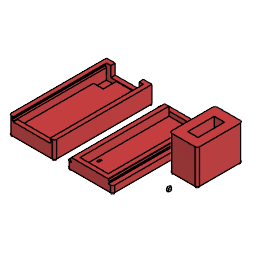
red_ducky-case (Autodesk Fusion 360 design; units mm, degrees)
part number: 2025-12-17-15-00-24-933
part number: 2025-12-19-11-25-16-273
Autodesk Fusion 360 part; units mm, degrees
note: some values were not read from the file. Chosen so that the rebuilt part matches the saved one: which face or edge a step refers to; which pieces of a blend or face edit are solid. Set by a fixed rule: which sketch regions a step uses.
sketch "Sketch1" plane through (0, 0, 0) normal (1, 0, 0) x (0, 1, 0)
  line L0 (-7.5042, 20.5557) -> (9.4958, 20.5557)
  line L1 (9.4958, 20.5557) -> (9.4958, -20.4443)
  line L2 (9.4958, -20.4443) -> (-7.5042, -20.4443)
  line L3 (-7.5042, -20.4443) -> (-7.5042, 20.5557)
  line L4 (-9.5042, 22.5557) -> (11.4958, 22.5557)
  line L5 (11.4958, 22.5557) -> (11.4958, -22.4443)
  line L6 (11.4958, -22.4443) -> (-9.5042, -22.4443)
  line L7 (-9.5042, -22.4443) -> (-9.5042, 22.5557)
  line L8 (-7.5042, 20.5557) -> (-3.0042, 20.5557)
  line L9 (-3.0042, 20.5557) -> (-3.0042, 14.5557)
  line L10 (-3.0042, 14.5557) -> (-7.5042, 14.5557)
  line L11 (-7.5042, 14.5557) -> (-7.5042, 20.5557)
  line L12 (9.4958, 20.5557) -> (4.9958, 20.5557)
  line L13 (4.9958, 20.5557) -> (4.9958, 14.5557)
  line L14 (4.9958, 14.5557) -> (9.4958, 14.5557)
  line L15 (9.4958, 14.5557) -> (9.4958, 20.5557)
  dimension "d1" = 17
  dimension "d2" = 41
  dimension "d3" = 45
  dimension "d4" = 21
  dimension "d5" = 2
  dimension "d6" = 2
  dimension "d8" = 6
  dimension "d9" = 4.5
  dimension "d10" = 6
  dimension "d11" = 4.5
  constraint horizontal L0
  constraint vertical L1
  constraint horizontal L2
  constraint vertical L3
  constraint horizontal L4
  constraint vertical L5
  constraint horizontal L6
  constraint vertical L7
  constraint horizontal L8
  constraint vertical L9
  constraint horizontal L10
  constraint vertical L11
  constraint horizontal L12
  constraint vertical L13
  constraint horizontal L14
  constraint vertical L15
  measures "d1" distance of L1 L3
  measures "d2" distance of L0 L2
  measures "d3" distance of L4.start L6.end
  measures "d4" distance of L4.start L4.end
  measures "d5" distance of L3 L7
  measures "d6" distance of L0 L4
  measures "d8" distance of L0.start L10.end
  measures "d9" distance of L9 L11
  measures "d10" distance of L0.end L14.end
  measures "d11" distance of L13 L15
extrude "Extrude1" add sketch "Sketch1" along normal blind 2 contours L0 L3 L8 L9 L10 L11 | L0 L1 L12 L13 L14 L15 makes body 1 at (0, -6.0042, 16.5557) makes body 2 at (0, 7.9958, 16.5557)
extrude "Extrude2" add sketch "Sketch1" along normal blind 4 contours L0 L1 L2 L3 L9 L10 L13 L14 bodies 1 2
extrude "Extrude3" add sketch "Sketch1" along normal blind 10.8 bodies 1
sketch "Sketch2" plane through (10.8, 0, 0) normal (1, 0, 0) x (0, 1, 0)
  line L0 (9.4958, 20.5557) -> (9.4958, -20.4443)
  line L1 (9.4958, -20.4443) -> (-7.5042, -20.4443)
  line L2 (-7.5042, -20.4443) -> (-7.5042, 20.5557)
  line L3 (-7.5042, 20.5557) -> (9.4958, 20.5557)
  line L4 (-9.5042, -22.4443) -> (11.4958, -22.4443)
  line L5 (11.4958, -22.4443) -> (11.4958, 22.5557)
  line L6 (11.4958, 22.5557) -> (-9.5042, 22.5557)
  line L7 (-9.5042, 22.5557) -> (-9.5042, -22.4443)
  line L8 (-6.5042, 22.5557) -> (8.4958, 22.5557)
  line L9 (8.4958, 22.5557) -> (8.4958, 20.5557)
  line L10 (8.4958, 20.5557) -> (-6.5042, 20.5557)
  line L11 (-6.5042, 20.5557) -> (-6.5042, 22.5557)
  line L12 (11.4958, 22.5557) -> (11.4958, -22.4443)
  dimension "d18" = 15
  dimension "d19" = 3
  constraint horizontal L8
  constraint vertical L9
  constraint horizontal L10
  constraint vertical L11
  constraint coincident L3 L9.end
  constraint coincident L6 L8.start
  measures "d18" distance of L9 L11
  measures "d19" distance of L9 L12
extrude "Extrude4" cut sketch "Sketch2" against normal blind 2 contours L0 L1 L2 L3 L4 L5 L6 L7 L9 L11 L12 | L3 L6 L8 L9 L10 L11 bodies 1
extrude "Extrude5" cut sketch "Sketch2" against normal blind 5 contours L3 L6 L8 L9 L10 L11 bodies 1
extrude "Extrude6" cut 1 faces at (5.8, 3.4958, 21.2224) along direction (-1, 0, 0) blind 2 on bodies 1 bodies 1
extrude "Extrude7" add 1 faces at (5.4667, -6.5042, 21.8891) along direction (0, 1, 0) blind 1 on bodies 1 bodies 1
extrude "Extrude8" add 1 faces at (7.1333, 8.4958, 21.8891) along direction (0, -1, 0) blind 1 on bodies 1 bodies 1
sketch "Sketch3" plane through (0, 0, -22.4443) normal (0, 0, -1) x (1, 0, 0)
  line L0 (8.8, -11.4958) -> (8.8, 9.5042)
  line L1 (8.8, 9.5042) -> (0, 9.5042)
  line L2 (0, 9.5042) -> (0, -11.4958)
  line L3 (0, -11.4958) -> (8.8, -11.4958)
  line L4 (8.8, 9.5042) -> (0, 9.5042)
  line L5 (0, 9.5042) -> (0, 7.5042)
  line L6 (0, 7.5042) -> (8.8, 7.5042)
  line L7 (8.8, 7.5042) -> (8.8, 9.5042)
  line L8 (8.8, -11.4958) -> (0, -11.4958)
  line L9 (0, -11.4958) -> (0, -9.4958)
  line L10 (0, -9.4958) -> (8.8, -9.4958)
  line L11 (8.8, -9.4958) -> (8.8, -11.4958)
  line L12 (8.8, 7.5042) -> (6.8, 7.5042)
  line L13 (6.8, 7.5042) -> (6.8, -9.4958)
  line L14 (6.8, -9.4958) -> (8.8, -9.4958)
  line L15 (8.8, -9.4958) -> (8.8, 7.5042)
  line L16 (8.05, 7.5042) -> (7.55, 7.5042)
  line L17 (7.5494, 8.0042) -> (8.05, 8.0042)
  line L18 (8.05, 8.0042) -> (8.55, 7.5042)
  line L19 (7.5494, 8.0042) -> (7.0494, 7.5042)
  line L20 (8.05, -9.4958) -> (7.55, -9.4958)
  line L21 (7.55, -9.9958) -> (8.05, -9.9958)
  line L22 (8.05, -9.9958) -> (8.5529, -9.4929)
  line L23 (7.55, -9.9958) -> (7.05, -9.4958)
  dimension "d30" = 2
  dimension "d31" = 2
  dimension "d32" = 2
  dimension "d33" = 0.5
  dimension "d36" = 0.5
  dimension "d39" = 45
  dimension "d40" = 45
  dimension "d41" = 45
  dimension "d42" = 45
  constraint horizontal L4
  constraint vertical L5
  constraint horizontal L6
  constraint vertical L7
  constraint coincident L2 L5.end
  constraint coincident L0.end L1.start
  constraint horizontal L8
  constraint vertical L9
  constraint horizontal L10
  constraint vertical L11
  constraint coincident L2 L9.end
  constraint coincident L0.start L3.end
  constraint horizontal L12
  constraint vertical L13
  constraint horizontal L14
  constraint vertical L15
  constraint coincident L10 L13.end
  constraint horizontal L16
  constraint horizontal L17
  constraint coincident L6 L16.start
  constraint coincident L6 L18.end
  constraint coincident L6 L19.end
  constraint horizontal L20
  constraint horizontal L21
  constraint coincident L14 L20.start
  constraint coincident L14 L23.end
  measures "d30" distance of L0.end L6.end
  measures "d31" distance of L0.start L10.end
  measures "d32" distance of L13 L15
  measures "d33" distance of L16.start L17.end
  measures "d36" distance of L20.start L21.end
  measures "d39" angle of L10 L22
  measures "d40" angle of L12 L18
  measures "d41" angle of L12 L19
  measures "d42" angle of L14 L23
extrude "Extrude9" cut sketch "Sketch3" against normal blind 2 contours L0 L6 L10 L12 L13 L14 L15 L16 L20 bodies 1
extrude "Extrude10" cut sketch "Sketch3" against normal blind 43 contours L10 L14 L20 L21 L22 L23 | L6 L12 L16 L17 L18 L19 bodies 1
extrude "Extrude11" add 1 faces at (3.8, -0.3375, 21.8891) along direction (1, 0, 0) blind 0.2 on bodies 1 bodies 1
sketch "Sketch4" plane through (0, 9.9958, 0) normal (0, -1, 0) x (1, 0, 0)
  line L0 (7.55, -22.4443) -> (8.05, -22.4443)
  line L1 (8.05, -22.4443) -> (8.05, 20.5557)
  line L2 (8.05, 20.5557) -> (7.55, 20.5557)
  line L3 (7.55, 20.5557) -> (7.55, -22.4443)
  line L4 (7.55, 20.5557) -> (8.05, 20.5557)
  line L5 (8.05, 20.5557) -> (8.05, 20.0557)
  line L6 (8.05, 20.0557) -> (7.55, 20.0557)
  line L7 (8.05, 20.0557) -> (8.05, 18.5557)
  line L8 (8.05, 18.5557) -> (7.55, 18.5557)
  line L9 (7.55, 18.5557) -> (7.55, 20.0557)
  dimension "d49" = 0.5
  dimension "d50" = 1.5
  constraint horizontal L4
  constraint vertical L5
  constraint horizontal L6
  constraint coincident L2.end L3.start
  constraint vertical L7
  constraint horizontal L8
  constraint vertical L9
  measures "d49" distance of L2.end L6.end
  measures "d50" distance of L6.end L8.end
extrude "Extrude12" cut sketch "Sketch4" against normal blind 1 contours L1 L2 L3 L4 L5 L6 bodies 1
chamfer "Chamfer1" distance 1.5 distance2 1 1 edges at (7.8, 9.9958, 20.0557) measured on face at (7.7167, 9.9958, -8.2776) on bodies 1
sketch "Sketch5" plane through (0, -8.0042, 0) normal (0, 1, 0) x (-1, 0, 0)
  line L0 (-8.05, -22.4443) -> (-7.5494, -22.4443)
  line L1 (-7.5494, -22.4443) -> (-7.5494, 20.5557)
  line L2 (-7.5494, 20.5557) -> (-8.05, 20.5557)
  line L3 (-8.05, 20.5557) -> (-8.05, -22.4443)
  line L4 (-8.05, 20.5557) -> (-7.5494, 20.5557)
  line L5 (-7.5494, 20.5557) -> (-7.5494, 20.0557)
  line L6 (-7.5494, 20.0557) -> (-8.05, 20.0557)
  line L7 (-8.05, 20.0557) -> (-8.05, 20.5557)
  line L8 (-8.05, 20.0557) -> (-7.5, 20.0557)
  line L9 (-7.5, 20.0557) -> (-7.5, 18.5557)
  line L10 (-7.5, 18.5557) -> (-8.05, 18.5557)
  line L11 (-8.05, 18.5557) -> (-8.05, 20.0557)
  dimension "d55" = 0.5
  dimension "d56" = 1.5
  constraint horizontal L4
  constraint vertical L5
  constraint horizontal L6
  constraint vertical L7
  constraint coincident L2.end L3.start
  constraint horizontal L8
  constraint vertical L9
  constraint horizontal L10
  constraint vertical L11
  measures "d55" distance of L2.end L6.end
  measures "d56" distance of L6.end L10.end
extrude "Extrude13" cut sketch "Sketch5" against normal blind 1 contours L1 L2 L3 L4 L5 L6 L7 L8 bodies 1
chamfer "Chamfer2" distance 1.5 distance2 1 1 edges at (7.7997, -8.0042, 20.0557) measured on face at (7.8831, -8.0042, -8.2776) on bodies 1
sketch "Sketch6" plane through (0, 0, 0) normal (1, 0, 0) x (0, 1, 0)
  line L0 (24.8147, 22.7428) -> (45.8147, 22.7428)
  line L1 (45.8147, 22.7428) -> (45.8147, -22.2572)
  line L2 (45.8147, -22.2572) -> (24.8147, -22.2572)
  line L3 (24.8147, -22.2572) -> (24.8147, 22.7428)
  dimension "d65" = 45
  dimension "d73" = 21
  constraint horizontal L0
  constraint vertical L1
  constraint horizontal L2
  constraint vertical L3
  measures "d65" distance of L0.start L2.end
  measures "d73" distance of L1 L3
extrude "Extrude16" add sketch "Sketch6" along normal blind 2 separate body makes body 3
sketch "Sketch7" plane through (2, 0, 0) normal (1, 0, 0) x (0, 1, 0)
  line L0 (24.8147, -22.2572) -> (45.8147, -22.2572)
  line L1 (45.8147, -22.2572) -> (45.8147, 22.7428)
  line L2 (45.8147, 22.7428) -> (24.8147, 22.7428)
  line L3 (24.8147, 22.7428) -> (24.8147, -22.2572)
  line L4 (24.8147, 22.7428) -> (45.8147, 22.7428)
  line L5 (45.8147, 22.7428) -> (45.8147, 20.7428)
  line L6 (45.8147, 20.7428) -> (24.8147, 20.7428)
  line L7 (24.8147, 20.7428) -> (24.8147, 22.7428)
  line L8 (45.8147, 22.7428) -> (43.8147, 22.7428)
  line L9 (43.8147, 22.7428) -> (43.8147, -22.2572)
  line L10 (43.8147, -22.2572) -> (45.8147, -22.2572)
  line L11 (45.8147, -22.2572) -> (45.8147, 22.7428)
  line L12 (24.8147, -22.2572) -> (45.8147, -22.2572)
  line L13 (45.8147, -22.2572) -> (45.8147, -20.2572)
  line L14 (45.8147, -20.2572) -> (24.8147, -20.2572)
  line L15 (24.8147, -20.2572) -> (24.8147, -22.2572)
  line L16 (24.8147, -22.2572) -> (26.8147, -22.2572)
  line L17 (26.8147, -22.2572) -> (26.8147, 23)
  line L18 (26.8147, 23) -> (24.8147, 23)
  line L19 (24.8147, 23) -> (24.8147, -22.2572)
  line L20 (26.8147, 20.7428) -> (28.8147, 20.7428)
  line L21 (28.8147, 20.7428) -> (28.8147, -22.2572)
  line L22 (28.8147, -22.2572) -> (26.8147, -22.2572)
  line L23 (26.8147, -22.2572) -> (26.8147, 20.7428)
  line L24 (43.8147, 20.7428) -> (41.8147, 20.7428)
  line L25 (41.8147, 20.7428) -> (41.8147, -22.2572)
  line L26 (41.8147, -22.2572) -> (43.8147, -22.2572)
  line L27 (43.8147, -22.2572) -> (43.8147, 20.7428)
  dimension "d76" = 2
  dimension "d77" = 2
  dimension "d78" = 2
  dimension "d79" = 2
  dimension "d80" = 2
  dimension "d81" = 2
  constraint horizontal L4
  constraint vertical L5
  constraint horizontal L6
  constraint vertical L7
  constraint coincident L2.end L3.start
  constraint horizontal L8
  constraint vertical L9
  constraint horizontal L10
  constraint vertical L11
  constraint coincident L0 L9.end
  constraint coincident L1.end L2.start
  constraint horizontal L12
  constraint vertical L13
  constraint horizontal L14
  constraint vertical L15
  constraint coincident L0.start L3.end
  constraint horizontal L16
  constraint vertical L17
  constraint horizontal L18
  constraint vertical L19
  constraint horizontal L20
  constraint vertical L21
  constraint horizontal L22
  constraint vertical L23
  constraint coincident L12 L21.end
  constraint coincident L17 L20.start
  constraint coincident L6 L20.start
  constraint horizontal L24
  constraint vertical L25
  constraint horizontal L26
  constraint vertical L27
  constraint coincident L0 L25.end
  constraint coincident L9 L24.start
  constraint coincident L6 L24.start
  measures "d76" distance of L2.end L6.end
  measures "d77" distance of L9 L11
  measures "d78" distance of L0.start L14.end
  measures "d79" distance of L17 L19
  measures "d80" distance of L17 L21
  measures "d81" distance of L9 L25
extrude "Extrude17" add sketch "Sketch7" along normal blind 2 contours L0 L3 L12 L14 L15 L16 L17 L19 L23 | L3 L6 L14 L17 L19 L23 | L2 L3 L4 L6 L7 L17 L19 | L2 L4 L6 L9 L17 L20 L24 | L0 L1 L9 L10 L11 L12 L13 L14 L27 | L1 L6 L9 L11 L14 L27 | L1 L2 L4 L5 L6 L8 L9 L11 bodies 3
extrude "Extrude18" add sketch "Sketch7" along normal blind 4 contours L0 L12 L14 L17 L21 L22 L23 | L0 L12 L14 L21 L25 | L6 L14 L17 L20 L21 L23 | L0 L9 L12 L14 L25 L26 L27 | L6 L9 L14 L24 L25 L27 bodies 3
sketch "Sketch8" plane through (0, 26.8147, 0) normal (0, -1, 0) x (1, 0, 0)
  line L0 (4, 20.7428) -> (4, -22.2572)
  line L1 (4, -22.2572) -> (6, -22.2572)
  line L2 (6, -22.2572) -> (6, 20.7428)
  line L3 (6, 20.7428) -> (4, 20.7428)
  line L4 (6, 20.7428) -> (5.75, 20.7428)
  line L5 (5.75, 20.7428) -> (5.75, -22.2572)
  line L6 (5.75, -22.2572) -> (6, -22.2572)
  line L7 (6, -22.2572) -> (6, 20.7428)
  line L8 (5.75, 20.7428) -> (5.25, 20.7428)
  line L9 (5.25, 20.7428) -> (5.25, -22.2572)
  line L10 (5.25, -22.2572) -> (5.75, -22.2572)
  line L11 (5.75, -22.2572) -> (5.75, 20.7428)
  line L12 (5.25, 20.7428) -> (4.75, 20.7428)
  line L13 (4.75, 20.7428) -> (4.75, -22.2572)
  line L14 (4.75, -22.2572) -> (5.25, -22.2572)
  line L15 (5.25, -22.2572) -> (5.25, 20.7428)
  line L16 (4, 20.7428) -> (4.25, 20.7428)
  line L17 (4.25, 20.7428) -> (4.25, -22.2572)
  line L18 (4.25, -22.2572) -> (4, -22.2572)
  line L19 (4, -22.2572) -> (4, 20.7428)
  dimension "d86" = 0.25
  dimension "d87" = 0.5
  dimension "d88" = 0.5
  dimension "d89" = 0.25
  constraint horizontal L4
  constraint vertical L5
  constraint horizontal L6
  constraint vertical L7
  constraint coincident L1 L5.end
  constraint coincident L2.end L3.start
  constraint horizontal L8
  constraint vertical L9
  constraint horizontal L10
  constraint vertical L11
  constraint coincident L1 L9.end
  constraint horizontal L12
  constraint vertical L13
  constraint horizontal L14
  constraint vertical L15
  constraint coincident L1 L13.end
  constraint horizontal L16
  constraint vertical L17
  constraint horizontal L18
  constraint vertical L19
  constraint coincident L1 L17.end
  constraint coincident L0.start L3.end
  measures "d86" distance of L5 L7
  measures "d87" distance of L5 L9
  measures "d88" distance of L9 L13
  measures "d89" distance of L17 L19
extrude "Extrude19" add sketch "Sketch8" along normal blind 0.5 contours L1 L3 L9 L12 L13 L14 L15 bodies 3
extrude "Extrude20" add sketch "Sketch8" along normal blind 0.5 contours L1 L3 L13 L17 | L1 L3 L5 L8 L9 L10 L11 L15 bodies 3
chamfer "Chamfer3" distance 0.5 angle 45 2 edges at (5.75, 26.3147, -0.7572) (4.25, 26.3147, -0.7572) on bodies 3
extrude "Extrude21" add 1 faces at (7.7167, 10.9958, 20.3891) along direction (0, -1, 0) blind 0.5 on bodies 1 bodies 1
delete_face "DeleteFace1" 5 faces at (7.8833, 10.829, 20.0557) (7.8833, 10.6623, 19.5558) (7.55, 10.1625, 19.7225) (7.7167, 10.4958, 20.3891) (8.05, 10.1625, 19.7225) on bodies 1
extrude "Extrude22" cut sketch "Sketch4" against normal blind 0.5 contours L1 L2 L3 L4 L5 L6 bodies 1
chamfer "Chamfer4" distance 1.5 distance2 0.5 1 edges at (7.8, 9.9958, 20.0557) measured on face at (7.7167, 9.9958, -8.2776) on bodies 1
delete_face "DeleteFace2" 5 faces at (8.05, -8.3375, 19.7225) (7.8831, -8.3375, 19.0559) (7.5494, -8.3375, 19.7225) (7.8831, -9.0042, 20.3891) (7.7163, -9.0041, 20.0557) on bodies 1
extrude "Extrude23" cut sketch "Sketch5" against normal blind 0.5 contours L1 L2 L3 L4 L5 L6 L7 L8 bodies 1
chamfer "Chamfer5" distance 1.5 distance2 0.5 1 edges at (7.7997, -8.0042, 20.0557) measured on face at (7.8831, -8.0042, -8.2776) on bodies 1
sketch "Sketch9" plane through (0, 26.3147, 0) normal (0, -1, 0) x (1, 0, 0)
  line L0 (4.75, 20.7428) -> (4.75, -22.2572)
  line L1 (4.75, -22.2572) -> (5.25, -22.2572)
  line L2 (5.25, -22.2572) -> (5.25, 20.7428)
  line L3 (5.25, 20.7428) -> (4.75, 20.7428)
  line L4 (4.75, 20.7428) -> (5.25, 20.7428)
  line L5 (5.25, 20.7428) -> (5.25, 19.2428)
  line L6 (5.25, 19.2428) -> (4.75, 19.2428)
  line L7 (4.75, 19.2428) -> (4.75, 20.7428)
  line L8 (4.75, 19.2428) -> (5.25, 19.2428)
  line L9 (5.25, 19.2428) -> (5.25, 18.7428)
  line L10 (5.25, 18.7428) -> (4.75, 18.7428)
  line L11 (4.75, 18.7428) -> (4.75, 19.2428)
  line L12 (4.75, 18.7428) -> (5.25, 18.7428)
  line L13 (5.25, 18.7428) -> (5.25, 17.2428)
  line L14 (5.25, 17.2428) -> (4.75, 17.2428)
  line L15 (4.75, 17.2428) -> (4.75, 18.7428)
  dimension "d105" = 1.5
  dimension "d106" = 0.5
  dimension "d107" = 1.5
  constraint horizontal L4
  constraint vertical L5
  constraint horizontal L6
  constraint vertical L7
  constraint coincident L0.start L3.end
  constraint horizontal L8
  constraint vertical L9
  constraint horizontal L10
  constraint vertical L11
  constraint horizontal L12
  constraint vertical L13
  constraint horizontal L14
  constraint vertical L15
  measures "d105" distance of L0.start L6.end
  measures "d106" distance of L6.end L10.end
  measures "d107" distance of L10.end L14.end
extrude "Extrude24" add sketch "Sketch9" along normal blind 0.5 contours L0 L2 L6 L8 L9 L10 L11 L12 bodies 3
chamfer "Chamfer6" distance 1.5 distance2 0.5 1 edges at (5, 26.3147, 18.7428) measured on face at (5.0833, 26.3147, -8.5905) on bodies 3
chamfer "Chamfer7" distance 1.5 distance2 0.5 1 edges at (5, 26.3147, 19.2428) measured on face at (5.0833, 26.3147, -9.0904) on bodies 3
sketch "Sketch10" plane through (0, 43.8147, 0) normal (0, 1, 0) x (-1, 0, 0)
  line L0 (-4, -22.2572) -> (-4, 20.7428)
  line L1 (-4, 20.7428) -> (-6, 20.7428)
  line L2 (-6, 20.7428) -> (-6, -22.2572)
  line L3 (-6, -22.2572) -> (-4, -22.2572)
  line L4 (-6, 20.7428) -> (-5.75, 20.7428)
  line L5 (-5.75, 20.7428) -> (-5.75, -22.2572)
  line L6 (-5.75, -22.2572) -> (-6, -22.2572)
  line L7 (-6, -22.2572) -> (-6, 20.7428)
  line L8 (-4, -22.2572) -> (-4.25, -22.2572)
  line L9 (-4.25, -22.2572) -> (-4.25, 20.7428)
  line L10 (-4.25, 20.7428) -> (-4, 20.7428)
  line L11 (-4, 20.7428) -> (-4, -22.2572)
  line L12 (-5.75, -22.2572) -> (-5.25, -22.2572)
  line L13 (-5.25, -22.2572) -> (-5.25, 20.7428)
  line L14 (-5.25, 20.7428) -> (-5.75, 20.7428)
  line L15 (-5.75, 20.7428) -> (-5.75, -22.2572)
  line L16 (-5.25, -22.2572) -> (-4.75, -22.2572)
  line L17 (-4.75, -22.2572) -> (-4.75, 20.7428)
  line L18 (-4.75, 20.7428) -> (-5.25, 20.7428)
  line L19 (-5.25, 20.7428) -> (-5.25, -22.2572)
  dimension "d114" = 0.25
  dimension "d115" = 0.25
  dimension "d116" = 0.5
  dimension "d117" = 0.5
  constraint horizontal L4
  constraint vertical L5
  constraint horizontal L6
  constraint vertical L7
  constraint coincident L3 L5.end
  constraint coincident L1.end L2.start
  constraint horizontal L8
  constraint vertical L9
  constraint horizontal L10
  constraint vertical L11
  constraint coincident L1 L9.end
  constraint coincident L0.start L3.end
  constraint horizontal L12
  constraint vertical L13
  constraint horizontal L14
  constraint vertical L15
  constraint coincident L1 L13.end
  constraint horizontal L16
  constraint vertical L17
  constraint horizontal L18
  constraint vertical L19
  constraint coincident L1 L17.end
  measures "d114" distance of L5 L7
  measures "d115" distance of L9 L11
  measures "d116" distance of L5 L13
  measures "d117" distance of L17 L19
extrude "Extrude25" add sketch "Sketch10" along normal blind 0.5 contours L1 L3 L9 L17 | L1 L3 L13 L16 L17 L18 L19 | L1 L3 L5 L12 L13 L14 L15 L19 bodies 3
chamfer "Chamfer8" distance 0.5 distance2 0.5 1 edges at (5.75, 44.3147, -0.7572) measured on face at (4.75, 44.3147, -7.9238) on bodies 3
chamfer "Chamfer9" distance 0.5 distance2 0.5 1 edges at (4.25, 44.3147, -0.7572) measured on face at (4.9167, 44.3147, -7.9238) on bodies 3
sketch "Sketch11" plane through (0, 44.3147, 0) normal (0, 1, 0) x (-1, 0, 0)
  line L0 (-4.75, -22.2572) -> (-4.75, 20.7428)
  line L1 (-4.75, 20.7428) -> (-5.25, 20.7428)
  line L2 (-5.25, 20.7428) -> (-5.25, -22.2572)
  line L3 (-5.25, -22.2572) -> (-4.75, -22.2572)
  line L4 (-5.25, 20.7428) -> (-4.75, 20.7428)
  line L5 (-4.75, 20.7428) -> (-4.75, 19.2428)
  line L6 (-4.75, 19.2428) -> (-5.25, 19.2428)
  line L7 (-5.25, 19.2428) -> (-5.25, 20.7428)
  line L8 (-5.25, 19.2428) -> (-4.75, 19.2428)
  line L9 (-4.75, 19.2428) -> (-4.75, 18.7428)
  line L10 (-4.75, 18.7428) -> (-5.25, 18.7428)
  line L11 (-5.25, 18.7428) -> (-5.25, 19.2428)
  line L12 (-5.25, 18.7428) -> (-4.75, 18.7428)
  line L13 (-4.75, 18.7428) -> (-4.75, 17.2428)
  line L14 (-4.75, 17.2428) -> (-5.25, 17.2428)
  line L15 (-5.25, 17.2428) -> (-5.25, 18.7428)
  dimension "d124" = 1.5
  dimension "d125" = 0.5
  dimension "d126" = 1.5
  constraint horizontal L4
  constraint vertical L5
  constraint horizontal L6
  constraint vertical L7
  constraint coincident L1.end L2.start
  constraint horizontal L8
  constraint vertical L9
  constraint horizontal L10
  constraint vertical L11
  constraint horizontal L12
  constraint vertical L13
  constraint horizontal L14
  constraint vertical L15
  measures "d124" distance of L1.end L6.end
  measures "d125" distance of L6.end L10.end
  measures "d126" distance of L10.end L14.end
extrude "Extrude26" add sketch "Sketch11" along normal blind 0.5 contours L0 L2 L10 L12 L13 L14 L15 | L0 L2 L6 L8 L9 L10 L11 L12 | L0 L1 L2 L4 L5 L6 L7 L8 bodies 3
chamfer "Chamfer10" distance 1.5 distance2 0.5 2 edges at (5, 44.8147, 17.2428) (5, 44.8147, 20.7428) measured on face at (5.0833, 44.8147, 18.4095) measured on face at (5.0833, 44.8147, 18.4095) on bodies 3
delete_face "DeleteFace3" 5 faces at (7.55, 10.1624, 19.7225) (7.7167, 10.1624, 19.0559) (8.05, 10.1624, 19.7225) (7.7167, 10.4958, 20.3891) (7.8833, 10.4957, 20.0557) on bodies 1
sketch "Sketch12" plane through (0, 9.9958, 0) normal (0, -1, 0) x (1, 0, 0)
  line L0 (7.55, 20.5557) -> (7.55, -22.4443)
  line L1 (7.55, -22.4443) -> (8.05, -22.4443)
  line L2 (8.05, -22.4443) -> (8.05, 20.5557)
  line L3 (8.05, 20.5557) -> (7.55, 20.5557)
  line L4 (7.55, 20.5557) -> (8.05, 20.5557)
  line L5 (8.05, 20.5557) -> (8.05, 19.0557)
  line L6 (8.05, 19.0557) -> (7.55, 19.0557)
  line L7 (7.55, 19.0557) -> (7.55, 20.5557)
  line L8 (7.55, 19.0557) -> (8.05, 19.0557)
  line L9 (8.05, 19.0557) -> (8.05, 18.4557)
  line L10 (8.05, 18.4557) -> (7.55, 18.4557)
  line L11 (7.55, 18.4557) -> (7.55, 19.0557)
  line L12 (7.55, 18.4557) -> (8.05, 18.4557)
  line L13 (8.05, 18.4557) -> (8.05, 16.9557)
  line L14 (8.05, 16.9557) -> (7.55, 16.9557)
  line L15 (7.55, 16.9557) -> (7.55, 18.4557)
  dimension "d131" = 1.5
  dimension "d132" = 0.6
  dimension "d133" = 1.5
  constraint horizontal L4
  constraint vertical L5
  constraint horizontal L6
  constraint vertical L7
  constraint coincident L2 L5.end
  constraint coincident L0.start L3.end
  constraint horizontal L8
  constraint vertical L9
  constraint horizontal L10
  constraint vertical L11
  constraint horizontal L12
  constraint vertical L13
  constraint horizontal L14
  constraint vertical L15
  measures "d131" distance of L0.start L6.end
  measures "d132" distance of L6.end L10.end
  measures "d133" distance of L10.end L14.end
extrude "Extrude27" cut sketch "Sketch12" against normal blind 0.5 contours L0 L2 L6 L8 L9 L10 L11 L12 bodies 1
chamfer "Chamfer11" distance 1.5 distance2 0.5 2 edges at (7.8, 9.9958, 18.4557) (7.8, 9.9958, 19.0557) measured on face at (7.7167, 9.9958, -8.8109) measured on face at (7.8833, 9.9958, 20.0557) on bodies 1
delete_face "DeleteFace4" 5 faces at (8.05, -8.1708, 19.7225) (7.8831, -8.1708, 19.0559) (7.5494, -8.1708, 19.7225) (7.8831, -8.5042, 20.3891) (7.7163, -8.5041, 20.0557) on bodies 1
sketch "Sketch13" plane through (0, -8.0042, 0) normal (0, 1, 0) x (-1, 0, 0)
  line L0 (-8.05, 20.5557) -> (-8.05, -22.4443)
  line L1 (-8.05, -22.4443) -> (-7.5494, -22.4443)
  line L2 (-7.5494, -22.4443) -> (-7.5494, 20.5557)
  line L3 (-7.5494, 20.5557) -> (-8.05, 20.5557)
  line L4 (-8.05, 20.5557) -> (-7.5494, 20.5557)
  line L5 (-7.5494, 20.5557) -> (-7.5494, 19.0557)
  line L6 (-7.5494, 19.0557) -> (-8.05, 19.0557)
  line L7 (-8.05, 19.0557) -> (-8.05, 20.5557)
  line L8 (-8.05, 19.0557) -> (-7.5494, 19.0557)
  line L9 (-7.5494, 19.0557) -> (-7.5494, 18.4557)
  line L10 (-7.5494, 18.4557) -> (-8.05, 18.4557)
  line L11 (-8.05, 18.4557) -> (-8.05, 19.0557)
  line L12 (-8.05, 18.4557) -> (-7.5494, 18.4557)
  line L13 (-7.5494, 18.4557) -> (-7.5494, 16.9557)
  line L14 (-7.5494, 16.9557) -> (-8.05, 16.9557)
  line L15 (-8.05, 16.9557) -> (-8.05, 18.4557)
  dimension "d138" = 1.5
  dimension "d139" = 0.6
  dimension "d140" = 1.5
  constraint horizontal L4
  constraint vertical L5
  constraint horizontal L6
  constraint vertical L7
  constraint coincident L0.start L3.end
  constraint horizontal L8
  constraint vertical L9
  constraint horizontal L10
  constraint vertical L11
  constraint horizontal L12
  constraint vertical L13
  constraint horizontal L14
  constraint vertical L15
  measures "d138" distance of L0.start L6.end
  measures "d139" distance of L6.end L10.end
  measures "d140" distance of L10.end L14.end
extrude "Extrude28" cut sketch "Sketch13" against normal blind 0.5 contours L0 L2 L6 L8 L9 L10 L11 L12 bodies 1
chamfer "Chamfer12" distance 1.5 distance2 0.5 2 edges at (7.7997, -8.0042, 19.0557) (7.7997, -8.0042, 18.4557) measured on face at (7.8831, -8.0042, 20.0557) measured on face at (7.7163, -8.0042, -8.8109) on bodies 1
fillet "Fillet1" radius 1 1 edges at (0, 11.4958, 0.0557) on bodies 1
fillet "Fillet2" radius 1 1 edges at (0, -9.5042, 0.0557) on bodies 1
fillet "Fillet3" radius 1 5 edges at (4.9, 11.4958, -22.4443) (0.2929, 11.2029, -22.4443) (0, 0.9958, -22.4443) (0.2929, -9.2113, -22.4443) (4.9, -9.5042, -22.4443) on bodies 1
fillet "Fillet4" radius 1 1 edges at (2, 24.8147, -22.2572) on bodies 3
fillet "Fillet5" radius 1 3 edges at (0, 35.8147, -22.2572) (0, 25.1076, -21.9643) (0, 24.8147, 0.7428) on bodies 3
fillet "Fillet6" radius 1 3 edges at (0, 45.8147, 0.7428) (0.2929, 45.8147, -21.9643) (2.5, 45.8147, -22.2572) on bodies 3
move_body "Move1" bodies 3 to x (-1, 0, 0) y (0, -1, 0) z (0, 0, 1) at (12.8, 36.3294, 0)
move_body "Move2" bodies 3 to x (1, 0, 0) y (0, 1, 0) z (0, 0, 1) at (0, 0, -0.2)
move_body "Move3" bodies 3 to x (1, 0, 0) y (0, 1, 0) z (0, 0, 1) at (0, 0, 0.023)
move_body "Move4" bodies 3 to x (1, 0, 0) y (0, 1, 0) z (0, 0, 1) at (0, -0.019, 0)
move_body "Move5" bodies 3 to x (1, 0, 0) y (0, 1, 0) z (0, 0, 1) at (0, 0, -0.01)
sketch "Sketch14" plane through (4, 0, 0) normal (1, 0, 0) x (0, 1, 0)
  line L0 (-3.0042, 20.5557) -> (-3.0042, 14.5557)
  line L1 (-3.0042, 14.5557) -> (-7.5042, 14.5557)
  line L2 (-7.5042, 14.5557) -> (-7.5042, -20.4443)
  line L3 (-7.5042, -20.4443) -> (9.4958, -20.4443)
  line L4 (9.4958, -20.4443) -> (9.4958, 14.5557)
  line L5 (9.4958, 14.5557) -> (4.9958, 14.5557)
  line L6 (4.9958, 14.5557) -> (4.9958, 20.5557)
  line L7 (4.9958, 20.5557) -> (7.4958, 20.5557)
  line L8 (7.4958, 20.5557) -> (7.4958, 22.5557)
  line L9 (7.4958, 22.5557) -> (-5.5042, 22.5557)
  line L10 (-5.5042, 22.5557) -> (-5.5042, 20.5557)
  line L11 (-5.5042, 20.5557) -> (-3.0042, 20.5557)
  line L12 (7.4958, 20.5557) -> (-5.5042, 20.5557)
  line L13 (-5.5042, 20.5557) -> (-5.5042, 22.5557)
  line L14 (-5.5042, 22.5557) -> (7.4958, 22.5557)
  line L15 (7.4958, 22.5557) -> (7.4958, 20.5557)
  constraint horizontal L12
  constraint vertical L13
  constraint horizontal L14
  constraint vertical L15
  constraint coincident L9.end L10.start
  constraint coincident L7.end L8.start
extrude "Extrude29" cut sketch "Sketch14" against normal blind 0.2 contours L0 L1 L2 L3 L4 L5 L6 L12 bodies 1
extrude "Extrude30" cut 1 faces at (3.8, 2.3291, -8.7776) along direction (-1, 0, 0) blind 0.5 on bodies 1 bodies 1
extrude "Extrude31" add 1 faces at (3.3, 2.3291, -8.7776) along direction (1, 0, 0) blind 0.4 on bodies 1 bodies 1
sketch "Sketch15" plane through (12.8, 0, 0) normal (1, 0, 0) x (0, 1, 0)
  line L0 (-8.5043, 22.5558) -> (-8.5043, -21.4442)
  line L1 (-8.5043, -21.4442) -> (10.4957, -21.4442)
  line L2 (10.4957, -21.4442) -> (10.4957, 22.5558)
  line L3 (10.4957, 22.5558) -> (-8.5043, 22.5558)
  line L4 (-8.5043, -21.4442) -> (10.4957, -21.4442)
  line L5 (10.4957, -21.4442) -> (10.4957, -20.4442)
  line L6 (10.4957, -20.4442) -> (-8.5043, -20.4442)
  line L7 (-8.5043, -20.4442) -> (-8.5043, -21.4442)
  line L8 (-8.5043, 22.5558) -> (10.4957, 22.5558)
  line L9 (10.4957, 22.5558) -> (10.4957, 20.5558)
  line L10 (10.4957, 20.5558) -> (-8.5043, 20.5558)
  line L11 (-8.5043, 20.5558) -> (-8.5043, 22.5558)
  line L12 (-8.5043, 22.5558) -> (-7.5043, 22.5558)
  line L13 (-7.5043, 22.5558) -> (-7.5043, -21.4442)
  line L14 (-7.5043, -21.4442) -> (-8.5043, -21.4442)
  line L15 (-8.5043, -21.4442) -> (-8.5043, 22.5558)
  line L16 (10.4957, 22.5558) -> (9.4957, 22.5558)
  line L17 (9.4957, 22.5558) -> (9.4957, -21.4442)
  line L18 (9.4957, -21.4442) -> (10.4957, -21.4442)
  line L19 (10.4957, -21.4442) -> (10.4957, 22.5558)
  line L20 (5.3957, -12.4442) -> (6.1957, -12.4442)
  line L21 (6.1957, -12.4442) -> (6.1957, -14.0442)
  line L22 (6.1957, -14.0442) -> (5.3957, -14.0442)
  line L23 (5.3957, -14.0442) -> (5.3957, -12.4442)
  dimension "d163" = 1
  dimension "d164" = 2
  dimension "d165" = 1
  dimension "d166" = 1
  dimension "d167" = 17
  dimension "d168" = 6.4
  dimension "d169" = 3.3
  dimension "d170" = 0.8
  dimension "d171" = 1.6
  constraint horizontal L4
  constraint vertical L5
  constraint horizontal L6
  constraint vertical L7
  constraint coincident L0.end L1.start
  constraint horizontal L8
  constraint vertical L9
  constraint horizontal L10
  constraint vertical L11
  constraint coincident L0.start L3.end
  constraint horizontal L12
  constraint vertical L13
  constraint horizontal L14
  constraint vertical L15
  constraint coincident L4 L13.end
  constraint horizontal L16
  constraint vertical L17
  constraint horizontal L18
  constraint vertical L19
  constraint coincident L4 L17.end
  constraint horizontal L20
  constraint vertical L21
  constraint horizontal L22
  constraint vertical L23
  measures "d163" distance of L0.end L6.end
  measures "d164" distance of L0.start L10.end
  measures "d165" distance of L13 L15
  measures "d166" distance of L17 L19
  measures "d167" distance of L13 L17
  measures "d168" distance of L6 L22
  measures "d169" distance of L17 L21
  measures "d170" distance of L21 L23
  measures "d171" distance of L20 L22
extrude "Extrude32" cut sketch "Sketch15" against normal blind 2 contours L20 L21 L22 L23 bodies 3
extrude "Extrude1'" add 1 faces at (12.1333, 6.1957, -12.9775) along direction (0, -1, 0) blind 0.8 separate body on bodies 3 makes body 4 in component "LED_hole"
extrude "Extrude2'" cut 1 faces at (10.8, 5.929, -12.9775) along direction (1, 0, 0) blind 0.5 on bodies 4 bodies 4 in component "LED_hole"
sketch "Sketch16" plane through (0, 0, 0) normal (0, 0, 1) x (1, 0, 0)
  line L0 (0.1176, 41.5067) -> (12.9176, 41.5067)
  line L1 (12.9176, 41.5067) -> (12.9176, 20.5067)
  line L2 (12.9176, 20.5067) -> (0.1176, 20.5067)
  line L3 (0.1176, 20.5067) -> (0.1176, 41.5067)
  dimension "d178" = 12.8
  dimension "d179" = 21
  constraint horizontal L0
  constraint vertical L1
  constraint horizontal L2
  constraint vertical L3
  measures "d178" distance of L1 L3
  measures "d179" distance of L0 L2
extrude "Extrude33" add sketch "Sketch16" along normal blind 2 separate body makes body 5
sketch "Sketch17" plane through (0, 0, 2) normal (0, 0, 1) x (-1, 0, 0)
  line L0 (-0.1176, -20.5067) -> (-12.9176, -20.5067)
  line L1 (-12.9176, -20.5067) -> (-12.9176, -41.5067)
  line L2 (-12.9176, -41.5067) -> (-0.1176, -41.5067)
  line L3 (-0.1176, -41.5067) -> (-0.1176, -20.5067)
  line L4 (-4.1676, -37.1067) -> (-8.8676, -37.1067)
  line L5 (-8.8676, -37.1067) -> (-8.8676, -24.9067)
  line L6 (-8.8676, -24.9067) -> (-4.1676, -24.9067)
  line L7 (-4.1676, -24.9067) -> (-4.1676, -37.1067)
  dimension "d182" = 4.7
  dimension "d183" = 12.2
  dimension "d184" = 4.05
  dimension "d185" = 4.4
  constraint horizontal L4
  constraint vertical L5
  constraint horizontal L6
  constraint vertical L7
  measures "d182" distance of L4.start L4.end
  measures "d183" distance of L4 L6
  measures "d184" distance of L3 L7
  measures "d185" distance of L0 L6
extrude "Extrude34" add sketch "Sketch17" along normal blind 14.8 bodies 5
fillet "Fillet7" radius 1 1 edges at (12.9176, 20.5067, 8.4) on bodies 5
fillet "Fillet8" radius 1 1 edges at (12.9176, 41.5067, 8.4) on bodies 5
fillet "Fillet9" radius 1 1 edges at (0.1176, 41.5067, 8.4) on bodies 5
fillet "Fillet10" radius 1 1 edges at (0.1176, 20.5067, 8.4) on bodies 5
fillet "Fillet11" radius 1 8 edges at (0.4104, 41.2138, 0) (6.5176, 41.5067, 0) (12.6247, 41.2138, 0) (12.9176, 31.0067, 0) (12.6247, 20.7996, 0) (6.5176, 20.5067, 0) (0.4104, 20.7996, 0) (0.1176, 31.0067, 0) on bodies 5
move_body "Move6" bodies 5 to x (1, 0, 0) y (0, -1, 0) z (0, 0, -1) at (0, 32.0134, 39)
move_body "Move7" bodies 5 to x (1, 0, 0) y (0, 1, 0) z (0, 0, 1) at (0, 0, 0.355)
move_body "Move8" bodies 5 to x (1, 0, 0) y (0, 1, 0) z (0, 0, 1) at (-0.118, 0, 0)
move_body "Move9" bodies 5 to x (1, 0, 0) y (0, 1, 0) z (0, 0, 1) at (0, 0, 17)
move_body "Move10" bodies 3 to x (0.819152, 0.573576, 0) y (-0.573576, 0.819152, 0) z (0, 0, 1) at (10.6245, -0.8982, 0)
move_body "Move11" bodies 3 to x (0.819152, -0.573576, 0) y (0.573576, 0.819152, 0) z (0, 0, 1) at (4.0294, 5.5073, 0)
move_body "Move12" bodies 3 to x (1, 0, 0) y (0, 1, 0) z (0, 0, 1) at (-12, 1, 0)
move_body "Move13" bodies 3 to x (1, 0, 0) y (0, 1, 0) z (0, 0, 1) at (-0.217, 0, 0)
move_body "Move14" bodies 3 to x (1, 0, 0) y (0, 1, 0) z (0, 0, 1) at (0, 0.323, 0)
move_body "Move15" bodies 1 to x (0, 0, 1) y (1, 0, 0) z (0, 1, 0) at (-12.4958, 12.9401, -22.4443)
move_body "Move16" bodies 1 to x (1, 0, 0) y (0, 1, 0) z (0, 0, 1) at (0, 0, 22.5)
move_body "Move17" bodies 3 to x (0, 0, -1) y (-1, 0, 0) z (0, 1, 0) at (16.2966, 12.9404, 12.8561)
move_body "Move18" bodies 5 to x (0, 1, 0) y (1, 0, 0) z (0, 0, -1) at (50.4929, 21.5071, 56.11)
move_body "Move19" bodies 5 to x (1, 0, 0) y (0, 1, 0) z (0, 0, 1) at (0, 0, 0.25)
move_body "Move20" bodies 5 to x (0, -1, 0) y (1, 0, 0) z (0, 0, 1) at (8.4929, 74.5062, 0)
component "LED_hole" placed x (1, 0, 0) y (0, 1, 0) z (0, 0, 1) at (0, 0, 0)
named bodies: "Case-bottom", "Case-top", "USB_cap"
